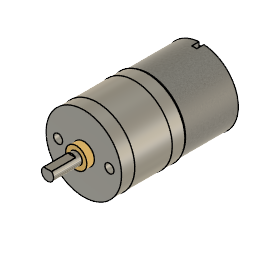
vac_v22 (Autodesk Fusion 360 archive; units mm, degrees)
design "CHR-GM25-BL2418"
Autodesk Fusion 360 part; units mm, degrees
sketch "Sketch1" plane through (0, 0, 0) normal (0, 1, 0) x (1, 0, 0)
  circle A0 centre (0, 0) radius 12.5
  line L0 (0, 0) -> (0, 12.5) construction
  point P0 (0, 12.5)
  dimension "d1" = 25
  constraint coincident A0.centre L0.start
  constraint coincident A0 P0
  constraint vertical L0
  constraint coincident P0 L0.end
  measures "d1" diameter of A0
extrude "Extrude1" add sketch "Sketch1" along normal blind 4.4 makes body 1
extrude "Extrude4" add 1 faces at (-3.3879, 4.4, 0.621) along direction (0, 1, 0) blind 12.4 separate body on bodies 1 makes body 2
extrude "Extrude5" add 1 faces at (-3.3879, 16.8, 0.621) along direction (0, 1, 0) blind 4.2 separate body on bodies 2 makes body 3
sketch "Sketch2" plane through (0, 21, 0) normal (0, 1, 0) x (-1, 0, 0)
  circle A0 centre (0, 0) radius 12.5
  circle A1 centre (0, 0) radius 12.2
  circle A2 centre (0, 0) radius 12.5
  dimension "d6" = 24.4
  constraint coincident A0.centre A1.centre
  measures "d6" diameter of A1
extrude "Extrude3" add sketch "Sketch2" along normal blind 18 separate body contours A1 makes body 4
fillet "Fillet1" radius 0.5 1 edges at (11.3744, 21, -4.4117) on bodies 4
sketch "Sketch3" plane through (0, 0, 0) normal (0, -1, 0) x (1, 0, 0)
  circle A0 centre (0, 0) radius 12.5
  circle A1 centre (0, 0) radius 3.5
  circle A2 centre (0, 0) radius 2
  dimension "d15" = 7
  dimension "d18" = 4
  constraint coincident A0.centre A1.centre
  constraint concentric A1 A2
  measures "d15" diameter of A1
  measures "d18" diameter of A2
extrude "Extrude6" add sketch "Sketch3" along normal blind 2.5 separate body contours A1 makes body 5
extrude "Extrude7" add sketch "Sketch3" along normal blind 12 separate body contours A2 makes body 6
sketch "Sketch4" plane through (0, -12, 0) normal (0, -1, 0) x (1, 0, 0)
  circle A0 centre (0, 0) radius 2
  circle A1 centre (0, 0) radius 2
  line L0 (-1.3229, 1.5) -> (1.3229, 1.5)
  dimension "d22" = 1.5
  constraint horizontal L0
  constraint coincident A1 L0.end
  constraint coincident A1 L0.start
  measures "d22" distance of L0 A0.centre
extrude "Extrude8" cut sketch "Sketch4" against normal blind 8 contours A0 A1 L0 picked at (-0.3643, 1.5583) bodies 1 6
sketch "Sketch5" plane through (0, 39, 0) normal (0, 1, 0) x (-1, 0, 0)
  circle A0 centre (0, 0) radius 12.2
  line L0 (-3.5, 10.2) -> (3.5, 10.2)
  line L1 (3.5, 10.2) -> (3.5, 7.2)
  line L2 (3.5, 7.2) -> (-3.5, 7.2)
  line L3 (-3.5, 7.2) -> (-3.5, 10.2)
  line L4 (0, 7.2) -> (0, 0)
  line L5 (0, 10.2) -> (0, 12.2) construction
  dimension "d25" = 7
  dimension "d26" = 3
  dimension "d27" = 5
  constraint horizontal L0
  constraint vertical L1
  constraint horizontal L2
  constraint vertical L3
  constraint midpoint L2 L4.start
  constraint coincident A0.centre L4.end
  constraint vertical L4
  constraint midpoint L0 L5.start
  constraint coincident A0 L5.end
  constraint perpendicular L0 L5
  measures "d25" distance of L0.start L0.end
  measures "d26" distance of L0.end L1.end
  measures "d27" distance of L4.start L5.end
extrude "Extrude9" add sketch "Sketch5" along normal blind 1 separate body contours L0 L1 L2 L3 makes body 7
sketch "Sketch6" plane through (0, 0, 0) normal (0, -1, 0) x (1, 0, 0)
  circle A0 centre (0, 0) radius 12.5
  line L0 (0, 0) -> (8.5, 0) construction
  line L1 (0, 0) -> (-8.5, 0) construction
  circle A1 centre (8.5, 0) radius 1.5
  circle A2 centre (-8.5, 0) radius 1.5
  dimension "d30" = 3
  dimension "d31" = 17
  constraint coincident A0.centre L0.start
  constraint horizontal L0
  constraint parallel L0 L1
  constraint equal L0 L1
  constraint coincident L0.end A1.centre
  constraint coincident L1.end A2.centre
  constraint equal A1 A2
  measures "d30" diameter of A1
  measures "d31" distance of L0.end L1.end
extrude "Extrude10" cut sketch "Sketch6" against normal through all contours A1 | A2 bodies 1 6
sketch "Sketch7" plane through (0, 39, 0) normal (0, 1, 0) x (-1, 0, 0)
  circle A0 centre (0, 0) radius 12.2
  circle A1 centre (0, 0) radius 3.2
  dimension "d34" = 6.4
  constraint coincident A0.centre A1.centre
  measures "d34" diameter of A1
extrude "Extrude11" add sketch "Sketch7" along normal blind 1.3 contours A1 bodies 4
sketch "Sketch8" plane through (0, 40.3, 0) normal (0, 1, 0) x (-1, 0, 0)
  circle A0 centre (0, 0) radius 3.2
  circle A1 centre (0, 0) radius 1
  dimension "d37" = 2
  constraint coincident A0.centre A1.centre
  measures "d37" diameter of A1
extrude "Extrude12" add sketch "Sketch8" along normal blind 1 separate body contours A1 makes body 8
sketch "Sketch9" plane through (0, 40, 0) normal (0, 1, 0) x (-1, 0, 0)
  line L0 (-3.5, 7.2) -> (3.5, 7.2)
  line L1 (3.5, 7.2) -> (3.5, 10.2)
  line L2 (3.5, 10.2) -> (-3.5, 10.2)
  line L3 (-3.5, 10.2) -> (-3.5, 7.2)
  line L4 (3.1, 9.8) -> (-3.1, 9.8)
  line L5 (-3.1, 9.8) -> (-3.1, 7.6)
  line L6 (-3.1, 7.6) -> (3.1, 7.6)
  line L7 (3.1, 7.6) -> (3.1, 9.8)
  dimension "d40" = -0.4
extrude "Extrude13" cut sketch "Sketch9" against normal blind 0.8 contours L4 L5 L6 L7 bodies 7
ref_plane "WorkPlane2" through (0, 31.2239, 12.2) normal (0, 0, 1) x (-1, 0, 0)
sketch "Sketch10" plane through (0, 31.2239, 12.2) normal (0, 0, 1) x (1, 0, 0)
  line L0 (12.2, 7.7761) -> (-12.2, 7.7761)
  line L1 (0, 0) -> (0, 7.7761) construction
  line L2 (0, 5.3761) -> (0.8, 5.3761)
  line L3 (0.8, 5.3761) -> (0.8, 7.7761)
  line L4 (0, 5.3761) -> (-0.8, 5.3761)
  line L5 (-0.8, 5.3761) -> (-0.8, 7.7761)
  dimension "d44" = 1.6
  dimension "d45" = 2.4
  constraint coincident L1.start origin
  constraint midpoint L0 L1.end
  constraint coincident L1 L2.start
  constraint perpendicular L1 L2
  constraint coincident L0 L3.end
  constraint perpendicular L0 L3
  constraint perpendicular L1 L4
  constraint coincident L0 L5.end
  constraint perpendicular L0 L5
  constraint equal L2 L4
  measures "d44" distance of L2.end L4.end
  measures "d45" distance of L2.end L3.end
extrude "Extrude14" cut sketch "Sketch10" against normal up to surface (2 mm away) bodies 4
equation "d11 = 21 mm - 4.4 mm - 4.2 mm"
named bodies: "Gearbox", "Motor"
